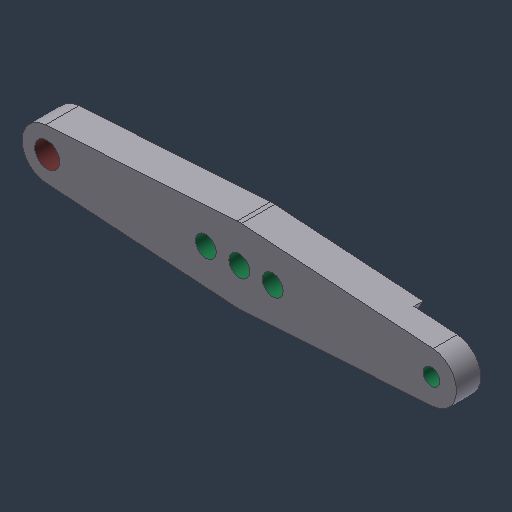
# Autodesk Inventor part: PLATE,ROCKER,ELEVATOR
Saved by Autodesk Inventor 2024.3 (Build 283343000, 343)
## iProperties
Category: _
Manager: _
ILogicPurgeVersion: 0.0.0.0
OnSaveVersion: 3.4.3.0
OnSaveAssembly: COREAutomationManager
Created: 2025-01-29
Part Number: PLATE,ROCKER,ELEVATOR
Checked By: 00
Engr Approved By: _
User Status: Work In Process
Material: Aluminum, 7075-T6
Description: STANDARD (mm)
Document SubType Name: Modeling
Mfg Approved By: John.Thibert
Designer: John.Thibert
Manufacturer: Standard
Standards Organization: Custom
Density: 2.81 g/cm^3
Appearance: Metal-AL-6061 (Flat)
Mass: 120.959 g
Surface Area: 128.954 cm^2
Volume: 43.0459 cm^3
CN_MASS: 0.12
CN_SERVICEABLE: _
FIRST_DESCRIPTION: _
SECOND_DESCRIPTION: _
THIRD_DESCRIPTION: _
ModelCat: Uncategorized
MaterialName: Aluminum, 7075-T6
Subject: _
Author: John.Thibert
Keywords: -
Revision Number: A
Autodesk Inventor part; units mm, degrees
ref_plane "YZ Plane" through (0, 0, 0) normal (1, 0, 0) x (0, 1, 0)
ref_plane "XZ Plane" through (0, 0, 0) normal (0, 1, 0) x (-1, 0, 0)
ref_plane "XY Plane" through (0, 0, 0) normal (0, 0, 1) x (1, 0, 0)
sketch "Sketch2" plane through (0, 0, 0) normal (0, 0, 1) x (1, 0, 0)
  line L0 (-73.6458, 9.5048) -> (-0.8277, 14.2605)
  arc A0 (0.8277, 14.2605) -> (-0.8277, 14.2605) centre (0, 1.5875) ccw
  line L1 (0.8277, 14.2605) -> (73.6458, 9.5048)
  arc A1 (73.6458, -9.5048) -> (73.6458, 9.5048) centre (73.025, 0) ccw
  line L2 (73.6458, -9.5048) -> (0.8277, -14.2605)
  arc A2 (-0.8277, -14.2605) -> (0.8277, -14.2605) centre (0, -1.5875) ccw
  line L3 (-0.8277, -14.2605) -> (-73.6458, -9.5048)
  arc A3 (-73.6458, 9.5048) -> (-73.6458, -9.5048) centre (-73.025, 0) ccw
  line L4 (-73.025, 0) -> (73.025, 0) construction
  line L5 (0, 20.0025) -> (0, -20.0025) construction
  line L6 (0, 1.5875) -> (0, -1.5875) construction
  point P0 (0, 0)
  point P1 (0, 0)
  dimension "d0" = 3.175
  dimension "d1" = 12.7
  dimension "d2" = 9.525
  dimension "d3" = 146.05
  constraints: 12 end point, 8 point on circle, 8 tangent, 4 centre point, 2 equal radius, 2 midpoint, 2 point on line, 1 coincident, 1 collinear, 1 horizontal
  measures "d0" distance of L6.start L6.end
  measures "d1" radius of A0
  measures "d2" radius of A1
  measures "d3" distance of L4.start L4.end
extrude "Extrusion1" add sketch "Sketch2" along normal mid plane 12.7
sketch "Sketch3" plane through (0, 0, 6.35) normal (0, 0, 1) x (1, 0, 0)
  line L0 (-12.7, 0) -> (12.7, 0) construction
  point P0 (0, 0)
  point P1 (0, 0)
  point P2 (0, 0)
  dimension "d6" = 25.4
  constraints: 4 coincident, 2 end point, 1 horizontal, 1 midpoint
  measures "d6" distance of L0.start L0.end
hole "Hole1" at (0, 0, 6.35) at (-12.7, 0, 6.35) at (12.7, 0, 6.35) direction (0, 0, -1) diameter 7.9502 end through all clearance for "F7 - SLIP FIT" size "5/16" standard "CL-DOWEL-IMP"
sketch "Sketch7" plane through (0, 0, 6.35) normal (0, 0, 1) x (1, 0, 0)
  arc A0 (-73.6458, 9.5048) -> (-73.6458, -9.5048) centre (-73.025, 0) ccw construction
  point P0 (0, 0)
  constraints: 1 coincident
hole "Hole4" at (-73.025, 0, 6.35) direction (0, 0, -1) diameter 9.525 end through all clearance for "H7 - STANDARD FIT" size "3/8" standard "CL-DOWEL-IMP"
sketch "Sketch9" plane through (0, 0, -6.35) normal (0, 0, -1) x (-1, 0, 0)
  circle A0 centre (73.025, 0) radius 4.7625 construction
  circle A1 centre (-12.7, 0) radius 3.9751 construction
  circle A2 centre (12.7, 0) radius 3.9751 construction
  circle A3 centre (0, 0) radius 3.9751 construction
  line L0 (-73.6458, -9.5048) -> (-0.8277, -14.2605) projected
  arc A4 (-0.8277, -14.2605) -> (0.8277, -14.2605) centre (0, -1.5875) ccw construction
  line L1 (0.8277, -14.2605) -> (73.6458, -9.5048) construction
  arc A5 (73.6458, -9.5048) -> (73.6458, 9.5048) centre (73.025, 0) ccw construction
  line L2 (73.6458, 9.5048) -> (0.8277, 14.2605) construction
  arc A6 (0.8277, 14.2605) -> (-0.8277, 14.2605) centre (0, 1.5875) ccw construction
  line L3 (-0.8277, 14.2605) -> (-73.6458, 9.5048) projected
  arc A7 (-73.6458, 9.5048) -> (-73.6458, -9.5048) centre (-73.025, 0) ccw projected
  arc A8 (-57.183, -10.5799) -> (-57.183, 10.5799) centre (-73.025, 0) ccw
  dimension "d48" = 19.05
  constraints: 9 centre point, 2 point on circle, 1 concentric
  measures "d48" radius of A8
extrude "Extrusion3" cut sketch "Sketch9" against normal blind 3.429
sketch "Sketch8" plane through (0, 0, 6.35) normal (0, 0, 1) x (1, 0, 0)
  arc A0 (73.6458, -9.5048) -> (73.6458, 9.5048) centre (73.025, 0) ccw construction
  point P0 (0, 0)
  point P1 (73.025, 0)
  constraints: 1 coincident
hole "Hole5" at (73.025, 0, 6.35) direction (0, 0, -1) diameter 6.35 end through all clearance for "F7 - SLIP FIT" size "1/4" standard "CL-DOWEL-IMP"
equation "\"d46\" = d0"
body "Solid1"
